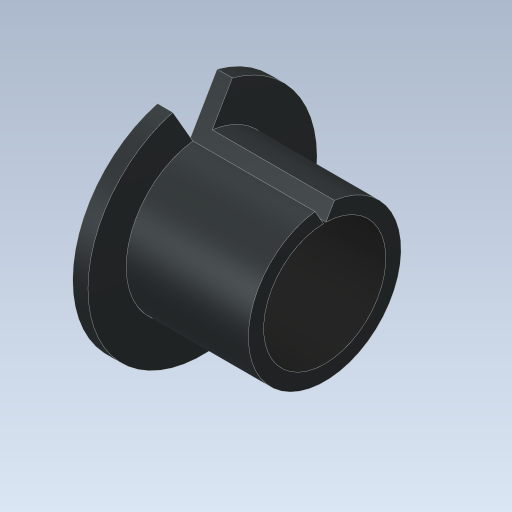
# Autodesk Inventor part: LFF-0808
Saved by Autodesk Inventor 2024 (Build 280153000, 153)
## iProperties
Created: 2023-09-30
Part Number: LFF-0808
Material: 鉄、鋳鉄
Catalog Web Link: www.cadenas.de
Description: Flange Bushings-LFF
Vendor: OILES
Document SubType Name: Modeling
Designer: psAdmin
Manufacturer: OILES
Mass: 2.42834 g
Surface Area: 7.72703 cm^2
Volume: 0.339628 cm^3
Density: 7.15 g/cm^3
Appearance: 鉄 ねずみ鋳鉄
Category: PARTsolutions
Company: OILES
PSOL_IDENT_0: {$CADENAS_DATA/23d-libs/oiles/multi_bearings/oiles_drymet_lf/flange_bushings_lff.prj},166 {VTYP=3D},
PSOL_IDENT_1: {NB=LFF-0808},{LINA=LFF-0808},{NN=Flange Bushings},{DATE=15.04.2019 22:54:28},{GEOMDATE=27.10.2016 0
PSOL_IDENT_2: 4:28:40},{VERSION=},{LINEID=180},{WBVAR=},{WBNUMERIC=}  {NB=LFF-0808},{LINA=LFF-0808},{KT=DUMMY},{OR
PSOL_IDENT_3: DERNO=LFF-0808},{S=8},{SRT=-0.025/-0.040},{H=10.0},{HRT=H7(+0.015/0)},{ID=8},{IDR=+0.065/0},{OD=10.0
PSOL_IDENT_4: },{IDT=+0.055/+0.025},{T=1.0},{TT=0/-0.025},{F=15},{R=1.500},{FDT=0/-0.8},{FT=1.0},{FTT=0/-0.15},{L=
PSOL_IDENT_5: 8},{LT=0/-0.3},{A=-},{AX=0.000},{B=-},{BC=0.000},{TE=-200~+280°C},{P=49.0N/mm2 (500kgf/cm2)},{V=0.65
PSOL_IDENT_6: m/s (39m/min)},{PV=3.60N/mm2•m/s (2,200kgf/cm2•m/min)},{AIT=The I.D. tolerance after press fitting i
PSOL_IDENT_7: s for reference only.},{AOT=Outer diameter is measrued by exclusive gauge.},{CAU=Please refer to cat
PSOL_IDENT_8: alog about detail.}
NB: LFF-0808
NN: Flange Bushings
NT: LFF
NBSYN: $ORDERNO.
LINA: LFF-0808
CATALOG: OILES CORPORATION
ORDERNO: LFF-0808
S: 8
SRT: -0.025/-0.040
H: 10
HRT: H7(+0.015/0)
ID: 8
IDR: +0.065/0
OD: 10
IDT: +0.055/+0.025
T: 1
TT: 0/-0.025
F: 15
FDT: 0/-0.8
FT: 1
FTT: 0/-0.15
L: 8
LT: 0/-0.3
TE: -200~+280°C
P: 49.0N/mm2 (500kgf/cm2)
V: 0.65m/s (39m/min)
PV: 3.60N/mm2•m/s (2,200kgf/cm2•m/min)
AIT: The I.D. tolerance after press fitting is for reference only.
AOT: Outer diameter is measrued by exclusive gauge.
CAU: Please refer to catalog about detail.
SUPPLIER: OILES
ARTICLENO: LFF-0808
BOMINFO: LFF-0808
CREATOR: CADENAS GmbH
Title: LFF-0808
Author: Cadenas PARTsolutions
Comments: LFF
Autodesk Inventor part; units mm, degrees
ref_plane "YZ Plane" through (0, 0, 0) normal (1, 0, 0) x (0, 1, 0)
ref_plane "XZ Plane" through (0, 0, 0) normal (0, 1, 0) x (-1, 0, 0)
ref_plane "XY Plane" through (0, 0, 0) normal (0, 0, 1) x (1, 0, 0)
sketch "Sketch_1" plane through (0, 0, 0) normal (0, 0, 1) x (1, 0, 0)
  line L0 (9, 0) -> (0, 0)
  line L1 (0, 4) -> (9, 4)
  line L2 (9, 4) -> (9, 5)
  line L3 (9, 5) -> (1, 5)
  line L4 (1, 5) -> (1, 7.5)
  line L5 (1, 7.5) -> (0, 7.5)
  line L6 (0, 7.5) -> (0, 4)
  constraints: 14 end point
revolve "Revolution1" add sketch "Sketch_1" angle 360 about axis through (9, 0, 0) along (1, 0, 0)
sketch "Sketch_3" plane through (0, 0, 0) normal (1, 0, 0) x (0, 1, 0)
  line L0 (10.4952, 3.83) -> (3.8614, 0)
  line L1 (3.8614, 0) -> (10.4952, -3.83)
  line L2 (10.4952, -3.83) -> (10.4952, 3.83)
  constraints: 6 end point
extrude "Extrusion1" cut sketch "Sketch_3" along normal blind 9
body "Solid1"
